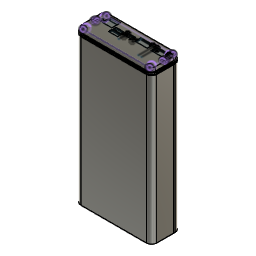
PowerBank65W v5 (Autodesk Fusion 360 design; units mm, degrees)
Autodesk Fusion 360 part; units mm, degrees
sketch "Sketch1" plane through (0, 0, 0) normal (0, 0, 1) x (1, 0, 0) in component "PWRBankModule"
  line L0 (3, 0) -> (78, 0)
  line L1 (81, 3) -> (81, 24)
  line L2 (78, 27) -> (3, 27)
  line L3 (0, 24) -> (0, 3)
  line L4 (2, 0) -> (2, 14.5)
  line L5 (2, 14.5) -> (0, 14.5)
  line L6 (0, 16.5) -> (2, 16.5)
  line L7 (2, 16.5) -> (2, 27)
  line L8 (79, 0) -> (79, 14.5)
  line L9 (79, 14.5) -> (81, 14.5)
  line L10 (81, 16.5) -> (79, 16.5)
  line L11 (79, 16.5) -> (79, 27)
  arc A0 (3, 27) -> (0, 24) centre (3, 24) ccw
  arc A1 (0, 3) -> (3, 0) centre (3, 3) ccw
  arc A2 (78, 0) -> (81, 3) centre (78, 3) ccw
  arc A3 (81, 24) -> (78, 27) centre (78, 24) ccw
  line L12 (82.5, 3) -> (82.5, 24)
  arc A4 (82.5, 24) -> (78, 28.5) centre (78, 24) ccw
  line L13 (78, 28.5) -> (3, 28.5)
  arc A5 (3, 28.5) -> (-1.5, 24) centre (3, 24) ccw
  line L14 (-1.5, 24) -> (-1.5, 3)
  arc A6 (-1.5, 3) -> (3, -1.5) centre (3, 3) ccw
  line L15 (3, -1.5) -> (78, -1.5)
  arc A7 (78, -1.5) -> (82.5, 3) centre (78, 3) ccw
  point P0 (81, 0)
  point P1 (0, 27)
  dimension "d1" = 81
  dimension "d2" = 1.5
  dimension "d3" = 77
  dimension "d4" = 2
  dimension "d5" = 2
  dimension "d6" = 2
  dimension "d7" = 2
  dimension "d8" = 2
  dimension "d9" = 14.5
  dimension "d10" = 14.5
  dimension "d11" = 27
  dimension "d50" = 3
  dimension "d51" = 3
  dimension "d52" = 3
  dimension "d53" = 3
  dimension "d54" = 12.5
  constraint horizontal L0
  constraint vertical L1
  constraint horizontal L2
  constraint vertical L3
  constraint coincident L0 L4.start
  constraint perpendicular L0 L4
  constraint coincident L3 L5.end
  constraint perpendicular L3 L5
  constraint coincident L3 L6.start
  constraint perpendicular L3 L6
  constraint coincident L2 L7.end
  constraint perpendicular L2 L7
  constraint coincident L0 L8.start
  constraint perpendicular L0 L8
  constraint coincident L1 L9.end
  constraint perpendicular L1 L9
  constraint coincident L1 L10.start
  constraint perpendicular L1 L10
  constraint coincident L2 L11.end
  constraint perpendicular L2 L11
  constraint coincident P1 L2
  constraint coincident P1 L3
  constraint tangent L2 A0
  constraint tangent L3 A0
  constraint coincident origin L0
  constraint coincident origin L3
  constraint tangent L0 A1
  constraint tangent L3 A1
  constraint coincident P0 L0
  constraint coincident P0 L1
  constraint tangent L0 A2
  constraint tangent L1 A2
  constraint tangent L1 A3
  constraint tangent L2 A3
  measures "d1" distance of origin P0
  measures "d3" distance of L4 L8
  measures "d4" distance of L4.end L5.end
  measures "d5" distance of L6.start L6.end
  measures "d6" distance of L10.start L10.end
  measures "d7" distance of L5 L6
  measures "d8" distance of L9 L10
  measures "d9" distance of L8.start L8.end
  measures "d10" distance of L4.start L4.end
  measures "d11" distance of origin P1
  measures "d50" radius of A0
  measures "d51" radius of A1
  measures "d52" radius of A2
  measures "d53" radius of A3
  measures "d54" distance of L2 L5
extrude "Extrude1" add sketch "Sketch1" along normal blind 3 contours L3 L4 L5 A1 | L1 L8 L9 A2 | L3 L6 L7 A0 | L1 L10 L11 A3 | L12 A4 L13 A5 L14 A6 L15 A7 makes body 1 in component "PWRBankModule"
sketch "Sketch2" plane through (0, 0, 3) normal (0, 0, 1) x (-1, 0, 0) in component "PWRBankModule"
  line L0 (-78, 0) -> (-3, 0)
  line L1 (0, -14.5) -> (0, -16.5)
  line L2 (-3, -27) -> (-78, -27)
  line L3 (-81, -16.5) -> (-81, -14.5)
  line L4 (-3, 1.5) -> (-78, 1.5)
  line L5 (-82.5, -3) -> (-82.5, -24)
  line L6 (-78, -28.5) -> (-3, -28.5)
  line L7 (1.5, -24) -> (1.5, -3)
  line L8 (-78, 0) -> (-3, 0) construction
  line L9 (-2, -0.1716) -> (-2, -14.5) construction
  line L10 (-2, -14.5) -> (0, -14.5) construction
  line L11 (0, -14.5) -> (0, -16.5) construction
  line L12 (0, -16.5) -> (-2, -16.5) construction
  line L13 (-2, -16.5) -> (-2, -26.8284) construction
  line L14 (-3, -27) -> (-78, -27) construction
  line L15 (-81, -16.5) -> (-81, -14.5) construction
  line L16 (-81, -14.5) -> (-79, -14.5) construction
  line L17 (-79, -14.5) -> (-79, -0.1716) construction
  line L18 (-79, -26.8284) -> (-79, -16.5) construction
  line L19 (-79, -16.5) -> (-81, -16.5) construction
  line L20 (-64, -23.1) -> (-78, -23.1)
  line L21 (-78, -23.1) -> (-78, -16.5)
  line L22 (-78, -16.5) -> (-64, -16.5)
  line L23 (-64, -16.5) -> (-64, -23.1)
  line L24 (-45.5, -23.1) -> (-59.5, -23.1)
  line L25 (-59.5, -23.1) -> (-59.5, -16.5)
  line L26 (-59.5, -16.5) -> (-45.5, -16.5)
  line L27 (-45.5, -16.5) -> (-45.5, -23.1)
  line L28 (-33, -20.5) -> (-42.5, -20.5)
  line L29 (-42.5, -20.5) -> (-42.5, -16.5)
  line L30 (-42.5, -16.5) -> (-33, -16.5)
  line L31 (-33, -16.5) -> (-33, -20.5)
  line L32 (-21, -19.3) -> (-30, -19.3)
  line L33 (-30, -19.3) -> (-30, -16)
  line L34 (-30, -16) -> (-21, -16)
  line L35 (-21, -16) -> (-21, -19.3)
  line L36 (-20.5, -15) -> (-31, -15)
  line L37 (-31, -15) -> (-31, -11)
  line L38 (-31, -11) -> (-20.5, -11)
  line L39 (-20.5, -11) -> (-20.5, -15)
  line L40 (-8, -26.5) -> (-19, -26.5)
  line L41 (-19, -26.5) -> (-19, -16.5)
  line L42 (-19, -16.5) -> (-8, -16.5)
  line L43 (-8, -16.5) -> (-8, -26.5)
  circle A0 centre (-5.5, -18.5) radius 1.75
  arc A1 (-3, -27) -> (-2, -26.8284) centre (-3, -24) ccw
  arc A2 (-79, -26.8284) -> (-78, -27) centre (-78, -24) ccw
  arc A3 (-78, 0) -> (-79, -0.1716) centre (-78, -3) ccw
  arc A4 (-2, -0.1716) -> (-3, 0) centre (-3, -3) ccw
  arc A5 (-78, 1.5) -> (-82.5, -3) centre (-78, -3) ccw
  arc A6 (-82.5, -24) -> (-78, -28.5) centre (-78, -24) ccw
  arc A7 (-3, -28.5) -> (1.5, -24) centre (-3, -24) ccw
  arc A8 (1.5, -3) -> (-3, 1.5) centre (-3, -3) ccw
  line L44 (-2, -0.1716) -> (-2, -14.5)
  line L45 (-2, -14.5) -> (0, -14.5)
  line L46 (0, -16.5) -> (-2, -16.5)
  line L47 (-2, -16.5) -> (-2, -26.8284)
  line L48 (-79, -26.8284) -> (-79, -16.5)
  line L49 (-79, -16.5) -> (-81, -16.5)
  line L50 (-81, -14.5) -> (-79, -14.5)
  line L51 (-79, -14.5) -> (-79, -0.1716)
  dimension "d14" = 81
  dimension "d15" = 14
  dimension "d16" = 14
  dimension "d17" = 4.5
  dimension "d18" = 6.6
  dimension "d20" = 3
  dimension "d21" = 48
  dimension "d22" = 9.5
  dimension "d23" = 60
  dimension "d24" = 9
  dimension "d25" = 3.3
  dimension "d26" = 4
  dimension "d27" = 60.5
  dimension "d28" = 10.5
  dimension "d29" = 4
  dimension "d30" = 73
  dimension "d31" = 11
  dimension "d32" = 10
  dimension "d33" = 75.5
  dimension "d34" = 3.5
  dimension "d35" = 8.6
  dimension "d38" = 1.5
  dimension "d39" = 0.5
  dimension "d40" = 2
  dimension "d55" = 6.6
  dimension "d56" = 4
  dimension "d57" = 6.6
  dimension "d58" = 2
  constraint horizontal L20
  constraint vertical L21
  constraint horizontal L22
  constraint vertical L23
  constraint horizontal L24
  constraint vertical L25
  constraint horizontal L26
  constraint vertical L27
  constraint horizontal L28
  constraint vertical L29
  constraint horizontal L30
  constraint vertical L31
  constraint horizontal L32
  constraint vertical L33
  constraint horizontal L34
  constraint vertical L35
  constraint horizontal L36
  constraint vertical L37
  constraint horizontal L38
  constraint vertical L39
  constraint horizontal L40
  constraint vertical L41
  constraint horizontal L42
  constraint vertical L43
  measures "d14" distance of L11 L15
  measures "d15" distance of L20.start L20.end
  measures "d16" distance of L24.start L24.end
  measures "d17" distance of L23 L25
  measures "d18" distance of L20.end L21.end
  measures "d20" distance of L15 L21
  measures "d21" distance of L15 L31
  measures "d22" distance of L28.start L28.end
  measures "d23" distance of L3 L35
  measures "d24" distance of L32.start L32.end
  measures "d25" distance of L32.end L33.end
  measures "d26" distance of L28.start L30.end
  measures "d27" distance of L15 L39
  measures "d28" distance of L36.start L36.end
  measures "d29" distance of L36.end L37.end
  measures "d30" distance of L15 L43
  measures "d31" distance of L40.start L40.end
  measures "d32" distance of L40.start L42.end
  measures "d33" distance of L15 A0.centre
  measures "d34" diameter of A0
  measures "d35" distance of L16 L20
  measures "d38" distance of L16 L34
  measures "d39" distance of L16 L36
  measures "d40" distance of L16 L42
  measures "d55" distance of L19 L24
  measures "d56" distance of L28 L49
  measures "d57" distance of L24.end L25.end
  measures "d58" distance of A0.centre L49
extrude "Extrude2" add sketch "Sketch2" along normal blind 1.5 contours L0 L1 L2 L3 A1 A2 A3 A4 L44 L45 L46 L47 L48 L49 L50 L51 | L4 L5 L6 L7 A5 A6 A7 A8 bodies 1 in component "PWRBankModule"
sketch "Sketch3" plane through (0, 0, 3) normal (0, 0, -1) x (1, 0, 0) in component "PWRBankModule"
  line L0 (45.5, -16.5) -> (59.5, -16.5)
  line L1 (59.5, -16.5) -> (59.5, -23.1)
  line L2 (59.5, -23.1) -> (45.5, -23.1)
  line L3 (45.5, -23.1) -> (45.5, -16.5)
  line L4 (33, -16.5) -> (42.5, -16.5)
  line L5 (42.5, -16.5) -> (42.5, -20.5)
  line L6 (42.5, -20.5) -> (33, -20.5)
  line L7 (33, -20.5) -> (33, -16.5)
  line L8 (64, -16.5) -> (78, -16.5)
  line L9 (78, -16.5) -> (78, -23.1)
  line L10 (78, -23.1) -> (64, -23.1)
  line L11 (64, -23.1) -> (64, -16.5)
  line L12 (21, -16) -> (30, -16)
  line L13 (30, -16) -> (30, -19.3)
  line L14 (30, -19.3) -> (21, -19.3)
  line L15 (21, -19.3) -> (21, -16)
  line L16 (20.5, -11) -> (31, -11)
  line L17 (31, -11) -> (31, -15)
  line L18 (31, -15) -> (20.5, -15)
  line L19 (20.5, -15) -> (20.5, -11)
  circle A0 centre (5.5, -18.5) radius 1.75
  line L20 (8, -16.5) -> (19, -16.5)
  line L21 (19, -16.5) -> (19, -26.5)
  line L22 (19, -26.5) -> (8, -26.5)
  line L23 (8, -26.5) -> (8, -16.5)
  line L24 (78, -23.1) -> (45.4821, -23.1)
  line L25 (45.4821, -23.1) -> (45.4821, -24.1)
  line L26 (45.4821, -24.1) -> (78, -24.1)
  line L27 (78, -24.1) -> (78, -23.1)
  line L28 (64, -23.1) -> (63, -23.1)
  line L29 (63, -23.1) -> (63, -6)
  line L30 (63, -6) -> (64, -6)
  line L31 (64, -6) -> (64, -23.1)
  line L32 (59.5, -23.1) -> (60.5, -23.1)
  line L33 (60.5, -23.1) -> (60.5, -6)
  line L34 (60.5, -6) -> (59.5, -6)
  line L35 (59.5, -6) -> (59.5, -23.1)
  line L36 (33, -20.5) -> (43.5, -20.5)
  line L37 (43.5, -20.5) -> (43.5, -21.5)
  line L38 (43.5, -21.5) -> (33, -21.5)
  line L39 (33, -21.5) -> (33, -20.5)
  line L40 (43.5, -20.5) -> (42.5, -20.5)
  line L41 (42.5, -20.5) -> (42.5, -16.5)
  line L42 (42.5, -16.5) -> (43.5, -16.5)
  line L43 (43.5, -16.5) -> (43.5, -20.5)
  line L44 (33, -16.5) -> (32, -16.5)
  line L45 (32, -16.5) -> (32, -10.9)
  line L46 (32, -10.9) -> (33, -10.9)
  line L47 (33, -10.9) -> (33, -16.5)
  line L48 (78, 0) -> (3, 0)
  arc A1 (3, 0) -> (2, -0.1716) centre (3, -3) ccw
  line L49 (2, -0.1716) -> (2, -14.5)
  line L50 (2, -14.5) -> (0, -14.5)
  line L51 (0, -14.5) -> (0, -16.5)
  line L52 (0, -16.5) -> (2, -16.5)
  line L53 (2, -16.5) -> (2, -26.8284)
  arc A2 (2, -26.8284) -> (3, -27) centre (3, -24) ccw
  line L54 (3, -27) -> (78, -27)
  arc A3 (78, -27) -> (79, -26.8284) centre (78, -24) ccw
  line L55 (79, -26.8284) -> (79, -16.5)
  line L56 (79, -16.5) -> (81, -16.5)
  line L57 (81, -16.5) -> (81, -14.5)
  line L58 (81, -14.5) -> (79, -14.5)
  line L59 (79, -14.5) -> (79, -0.1716)
  arc A4 (79, -0.1716) -> (78, 0) centre (78, -3) ccw
  dimension "d44" = 1
  dimension "d45" = 1
  dimension "d46" = 1
  dimension "d47" = 1
  dimension "d48" = 1
  dimension "d49" = 1
  constraint horizontal L24
  constraint vertical L25
  constraint horizontal L26
  constraint vertical L27
  constraint coincident L9.end L10.start
  constraint horizontal L28
  constraint vertical L29
  constraint horizontal L30
  constraint vertical L31
  constraint coincident L10.end L11.start
  constraint horizontal L32
  constraint vertical L33
  constraint horizontal L34
  constraint vertical L35
  constraint coincident L1.end L2.start
  constraint horizontal L36
  constraint vertical L37
  constraint horizontal L38
  constraint vertical L39
  constraint coincident L6.end L7.start
  constraint horizontal L40
  constraint vertical L41
  constraint horizontal L42
  constraint vertical L43
  constraint coincident L4.end L5.start
  constraint horizontal L44
  constraint vertical L45
  constraint horizontal L46
  constraint vertical L47
  constraint coincident L4.start L7.end
  measures "d44" distance of L9.end L26.end
  measures "d45" distance of L29.end L30.end
  measures "d46" distance of L33.end L34.end
  measures "d47" distance of L36.end L37.end
  measures "d48" distance of L4.end L42.end
  measures "d49" distance of L4.start L44.end
sketch "Sketch1 (2)" plane through (0, 0, 0) normal (0, 0, 1) x (1, 0, 0) in component "ButtLid"
  line L0 (3, -1.5) -> (78, -1.5) construction
  arc A0 (78, -1.5) -> (82.5, 3) centre (78, 3) ccw construction
  line L1 (82.5, 3) -> (82.5, 24) construction
  arc A1 (82.5, 24) -> (78, 28.5) centre (78, 24) ccw construction
  line L2 (78, 28.5) -> (3, 28.5) construction
  arc A2 (3, 28.5) -> (-1.5, 24) centre (3, 24) ccw construction
  line L3 (-1.5, 24) -> (-1.5, 3) construction
  arc A3 (-1.5, 3) -> (3, -1.5) centre (3, 3) ccw construction
  arc A4 (3, 28.6) -> (-1.6, 24) centre (3, 24) ccw
  line L4 (-1.6, 24) -> (-1.6, 3)
  arc A5 (-1.6, 3) -> (3, -1.6) centre (3, 3) ccw
  line L5 (3, -1.6) -> (78, -1.6)
  arc A6 (78, -1.6) -> (82.6, 3) centre (78, 3) ccw
  line L6 (82.6, 3) -> (82.6, 24)
  arc A7 (82.6, 24) -> (78, 28.6) centre (78, 24) ccw
  line L7 (78, 28.6) -> (3, 28.6)
  arc A8 (3, 30) -> (-3, 24) centre (3, 24) ccw
  line L8 (-3, 24) -> (-3, 3)
  arc A9 (-3, 3) -> (3, -3) centre (3, 3) ccw
  line L9 (3, -3) -> (78, -3)
  arc A10 (78, -3) -> (84, 3) centre (78, 3) ccw
  line L10 (84, 3) -> (84, 24)
  arc A11 (84, 24) -> (78, 30) centre (78, 24) ccw
  line L11 (78, 30) -> (3, 30)
  line L12 (84, 22) -> (82.6, 22)
  line L13 (82.6, 21) -> (81.1, 21)
  line L14 (81.1, 21) -> (81.1, 23)
  line L15 (81.1, 23) -> (82.5, 23)
  line L16 (82.5, 23) -> (82.5, 22)
  line L17 (82.5, 22) -> (82.6, 22)
  line L18 (-1.6, 22) -> (-3, 22)
  line L19 (-1.6, 22) -> (-1.5, 22)
  line L20 (-1.5, 22) -> (-1.5, 23)
  line L21 (-1.5, 23) -> (-0.1, 23)
  line L22 (-0.1, 23) -> (-0.1, 21)
  line L23 (-0.1, 21) -> (-1.6, 21)
  dimension "d59" = 0.1
  dimension "d60" = 1.5
  dimension "d61" = 1
  dimension "d62" = 2
  dimension "d63" = 1.5
  dimension "d64" = 0.1
  dimension "d65" = 25
  dimension "d70" = 1.5
  dimension "d71" = 2
  dimension "d72" = 1
  dimension "d73" = 0.1
  dimension "d74" = 25
  constraint coincident L6 L12.end
  constraint perpendicular L6 L12
  constraint coincident L6 L13.start
  constraint perpendicular L1 L13
  constraint perpendicular L13 L14
  constraint perpendicular L14 L15
  constraint perpendicular L15 L16
  constraint perpendicular L6 L17
  constraint coincident L4 L18.start
  constraint coincident L8 L18.end
  constraint perpendicular L8 L18
  constraint perpendicular L3 L19
  constraint perpendicular L18 L20
  constraint perpendicular L3 L21
  constraint perpendicular L21 L22
  constraint coincident L4 L23.end
  constraint perpendicular L4 L23
  measures "d61" distance of L15.end L16.end
  measures "d62" distance of L13.end L14.end
  measures "d63" distance of L13.start L13.end
  measures "d64" distance of L6 L16
  measures "d65" distance of L9 L12
  measures "d70" distance of L22.end L23.end
  measures "d71" distance of L21.end L22.end
  measures "d72" distance of L19.end L20.end
  measures "d73" distance of L18.start L19.end
  measures "d74" distance of L9 L18
extrude "Extrude1'" add sketch "Sketch1 (2)" against normal blind 170 separate body contours L4 L19 L20 L21 L22 L23 | L4 A5 L5 A6 L6 L8 A9 L9 A10 L10 L12 L18 | L6 L13 L14 L15 L16 L17 makes body 2 in component "ButtLid"
sketch "Sketch2 (2)" plane through (0, 0, 0) normal (0, 0, 1) x (-1, 0, 0) in component "ButtLid"
  line L0 (1.5, -22) -> (3, -22)
  line L1 (3, -22) -> (3, -3)
  arc A0 (3, -3) -> (-3, 3) centre (-3, -3) ccw
  line L2 (-3, 3) -> (-78, 3)
  arc A1 (-78, 3) -> (-84, -3) centre (-78, -3) ccw
  line L3 (-84, -3) -> (-84, -22)
  line L4 (-84, -22) -> (-82.5, -22)
  line L5 (-82.5, -22) -> (-82.5, -23)
  line L6 (-82.5, -23) -> (-81.1, -23)
  line L7 (-81.1, -23) -> (-81.1, -21)
  line L8 (-81.1, -21) -> (-82.6, -21)
  line L9 (-82.6, -21) -> (-82.6, -3)
  arc A2 (-78, 1.6) -> (-82.6, -3) centre (-78, -3) ccw
  line L10 (-78, 1.6) -> (-3, 1.6)
  arc A3 (1.6, -3) -> (-3, 1.6) centre (-3, -3) ccw
  line L11 (1.6, -3) -> (1.6, -21)
  line L12 (1.6, -21) -> (0.1, -21)
  line L13 (0.1, -21) -> (0.1, -23)
  line L14 (0.1, -23) -> (1.5, -23)
  line L15 (1.5, -23) -> (1.5, -22)
  line L16 (-82.6, -17.5) -> (-79, -17.5)
  line L17 (-79, -17.5) -> (-79, -16.5)
  line L18 (-79, -16.5) -> (-81, -16.5)
  line L19 (-81, -16.5) -> (-81, -14.5)
  line L20 (-81, -14.5) -> (-79, -14.5)
  line L21 (-79, -14.5) -> (-79, -13.5)
  line L22 (-79, -13.5) -> (-82.6, -13.5)
  line L23 (1.6, -17.5) -> (-2, -17.5)
  line L24 (-2, -17.5) -> (-2, -16.5)
  line L25 (-2, -16.5) -> (0, -16.5)
  line L26 (0, -16.5) -> (0, -14.5)
  line L27 (0, -14.5) -> (-2, -14.5)
  line L28 (-2, -14.5) -> (-2, -13.5)
  line L29 (-2, -13.5) -> (1.6, -13.5)
  point P0 (-79, -16.5)
  point P1 (-81, -16.5)
  point P2 (-81, -14.5)
  point P3 (-79, -14.5)
  point P4 (0, -14.5)
  point P5 (-2, -14.5)
  point P6 (-2, -16.5)
  point P7 (0, -16.5)
  dimension "d77" = 1
  dimension "d78" = 1
  dimension "d79" = 1
  dimension "d80" = 1
  constraint coincident L9 L16.start
  constraint perpendicular L9 L16
  constraint coincident P0 L17.end
  constraint coincident P1 L18.end
  constraint coincident P2 L19.end
  constraint coincident P3 L20.end
  constraint perpendicular L20 L21
  constraint coincident L9 L22.end
  constraint perpendicular L9 L22
  constraint coincident L11 L23.start
  constraint perpendicular L11 L23
  constraint coincident P6 L24.end
  constraint coincident P7 L25.end
  constraint coincident P4 L26.end
  constraint coincident P5 L27.end
  constraint perpendicular L27 L28
  constraint coincident L11 L29.end
  constraint perpendicular L11 L29
  measures "d77" distance of L16.end P0
  measures "d78" distance of P3 L21.end
  measures "d79" distance of P5 L28.end
  measures "d80" distance of L23.end P6
extrude "Extrude2'" add sketch "Sketch2 (2)" against normal blind 28 contours L11 L23 L24 L25 L26 L27 L28 L29 | L9 L16 L17 L18 L19 L20 L21 L22 bodies 2 in component "ButtLid"
sketch "Sketch3 (2)" plane through (0, 0, 0) normal (0, 0, 1) x (-1, 0, 0) in component "ButtLid"
  line L0 (1.5, -22) -> (3, -22)
  line L1 (3, -22) -> (3, -3)
  arc A0 (3, -3) -> (-3, 3) centre (-3, -3) ccw
  line L2 (-3, 3) -> (-78, 3)
  arc A1 (-78, 3) -> (-84, -3) centre (-78, -3) ccw
  line L3 (-84, -3) -> (-84, -22)
  line L4 (-84, -22) -> (-82.5, -22)
  line L5 (-82.5, -22) -> (-82.5, -23)
  line L6 (-82.5, -23) -> (-81.1, -23)
  line L7 (-81.1, -23) -> (-81.1, -21)
  line L8 (-81.1, -21) -> (-82.6, -21)
  line L9 (-82.6, -21) -> (-82.6, -17.5)
  line L10 (-82.6, -17.5) -> (-79, -17.5)
  line L11 (-79, -17.5) -> (-79, -16.5)
  line L12 (-79, -16.5) -> (-81, -16.5)
  line L13 (-81, -16.5) -> (-81, -14.5)
  line L14 (-81, -14.5) -> (-79, -14.5)
  line L15 (-79, -14.5) -> (-79, -13.5)
  line L16 (-79, -13.5) -> (-82.6, -13.5)
  line L17 (-82.6, -13.5) -> (-82.6, -3)
  arc A2 (-78, 1.6) -> (-82.6, -3) centre (-78, -3) ccw
  line L18 (-78, 1.6) -> (-3, 1.6)
  arc A3 (1.6, -3) -> (-3, 1.6) centre (-3, -3) ccw
  line L19 (1.6, -3) -> (1.6, -13.5)
  line L20 (1.6, -13.5) -> (-2, -13.5)
  line L21 (-2, -13.5) -> (-2, -14.5)
  line L22 (-2, -14.5) -> (0, -14.5)
  line L23 (0, -14.5) -> (0, -16.5)
  line L24 (0, -16.5) -> (-2, -16.5)
  line L25 (-2, -16.5) -> (-2, -17.5)
  line L26 (-2, -17.5) -> (1.6, -17.5)
  line L27 (1.6, -17.5) -> (1.6, -21)
  line L28 (1.6, -21) -> (0.1, -21)
  line L29 (0.1, -21) -> (0.1, -23)
  line L30 (0.1, -23) -> (1.5, -23)
  line L31 (1.5, -23) -> (1.5, -22)
  line L32 (-82.6, -13.5) -> (-79, -13.5)
  line L33 (-79, -13.5) -> (-79, -23)
  line L34 (-79, -23) -> (-82.6, -23)
  line L35 (-82.6, -23) -> (-82.6, -13.5)
  line L36 (1.6, -13.5) -> (-2, -13.5)
  line L37 (-2, -13.5) -> (-2, -23)
  line L38 (-2, -23) -> (1.6, -23)
  line L39 (1.6, -23) -> (1.6, -13.5)
  dimension "d83" = 3.6
  dimension "d84" = 3.6
  constraint horizontal L32
  constraint vertical L33
  constraint horizontal L34
  constraint vertical L35
  constraint coincident L16.end L17.start
  constraint horizontal L36
  constraint vertical L37
  constraint horizontal L38
  constraint vertical L39
  constraint coincident L19.end L20.start
  constraint coincident L6.end L34
  constraint coincident L29.end L38
  measures "d83" distance of L33.end L34.end
  measures "d84" distance of L37.end L38.end
extrude "Extrude3" cut sketch "Sketch3 (2)" against normal blind 4.6 contours L0 L28 L29 L30 L31 L38 L39 | L20 L21 L22 L23 L24 L25 L26 L36 L37 L39 | L4 L5 L6 L7 L8 L34 L35 | L10 L11 L12 L13 L14 L15 L16 L32 L33 L35 bodies 2 in component "ButtLid"
sketch "Sketch4" plane through (0, 0, -170) normal (0, 0, -1) x (1, 0, 0) in component "ButtLid"
  line L0 (-3, -22) -> (-1.5, -22)
  line L1 (-1.5, -22) -> (-1.5, -23)
  line L2 (-1.5, -23) -> (-0.1, -23)
  line L3 (-0.1, -23) -> (-0.1, -21)
  line L4 (-0.1, -21) -> (-1.6, -21)
  line L5 (-1.6, -21) -> (-1.6, -3)
  arc A0 (3, 1.6) -> (-1.6, -3) centre (3, -3) ccw
  line L6 (3, 1.6) -> (78, 1.6)
  arc A1 (82.6, -3) -> (78, 1.6) centre (78, -3) ccw
  line L7 (82.6, -3) -> (82.6, -21)
  line L8 (82.6, -21) -> (81.1, -21)
  line L9 (81.1, -21) -> (81.1, -23)
  line L10 (81.1, -23) -> (82.5, -23)
  line L11 (82.5, -23) -> (82.5, -22)
  line L12 (82.5, -22) -> (84, -22)
  line L13 (84, -22) -> (84, -3)
  arc A2 (84, -3) -> (78, 3) centre (78, -3) ccw
  line L14 (78, 3) -> (3, 3)
  arc A3 (3, 3) -> (-3, -3) centre (3, -3) ccw
  line L15 (-3, -3) -> (-3, -22)
  line L16 (-1.6, -21) -> (-0.1, -21)
  line L17 (-0.1, -21) -> (-0.1, -23)
  line L18 (-0.1, -23) -> (-1.6, -23)
  line L19 (-1.6, -23) -> (-1.6, -21)
  line L20 (82.6, -21) -> (81.1, -21)
  line L21 (81.1, -21) -> (81.1, -23)
  line L22 (81.1, -23) -> (82.6, -23)
  line L23 (82.6, -23) -> (82.6, -21)
  constraint horizontal L16
  constraint vertical L17
  constraint horizontal L18
  constraint vertical L19
  constraint coincident L2.end L3.start
  constraint coincident L4.end L5.start
  constraint horizontal L20
  constraint vertical L21
  constraint horizontal L22
  constraint vertical L23
  constraint coincident L9.end L10.start
  constraint coincident L7.end L8.start
extrude "Extrude4" cut sketch "Sketch4" against normal blind 1.6 contours L0 L1 L2 L3 L4 L16 L17 L18 L19 | L8 L9 L10 L11 L12 L20 L21 L22 L23 bodies 2 in component "ButtLid"
sketch "Sketch1 (3)" plane through (0, 0, 0) normal (0, 0, -1) x (1, 0, 0) in component "TopLid"
  arc A0 (3, 0) -> (2, -0.1716) centre (3, -3) ccw
  line L0 (3, 0) -> (78, 0)
  arc A1 (79, -0.1716) -> (78, 0) centre (78, -3) ccw
  line L1 (79, -0.1716) -> (79, -14.5)
  line L2 (79, -14.5) -> (81, -14.5)
  line L3 (81, -14.5) -> (81, -16.5)
  line L4 (81, -16.5) -> (79, -16.5)
  line L5 (79, -16.5) -> (79, -26.8284)
  arc A2 (78, -27) -> (79, -26.8284) centre (78, -24) ccw
  line L6 (78, -27) -> (3, -27)
  arc A3 (2, -26.8284) -> (3, -27) centre (3, -24) ccw
  line L7 (2, -26.8284) -> (2, -16.5)
  line L8 (2, -16.5) -> (0, -16.5)
  line L9 (0, -16.5) -> (0, -14.5)
  line L10 (0, -14.5) -> (2, -14.5)
  line L11 (2, -14.5) -> (2, -0.1716)
  arc A4 (82.5, -3) -> (78, 1.5) centre (78, -3) ccw
  line L12 (78, 1.5) -> (3, 1.5)
  arc A5 (3, 1.5) -> (-1.5, -3) centre (3, -3) ccw
  line L13 (-1.5, -3) -> (-1.5, -24)
  arc A6 (-1.5, -24) -> (3, -28.5) centre (3, -24) ccw
  line L14 (3, -28.5) -> (78, -28.5)
  arc A7 (78, -28.5) -> (82.5, -24) centre (78, -24) ccw
  line L15 (82.5, -24) -> (82.5, -3)
  line L16 (78, -28.5) -> (3, -28.5) construction
  arc A8 (-1.5, -24) -> (3, -28.5) centre (3, -24) ccw construction
  line L17 (-1.5, -24) -> (-1.5, -3) construction
  line L18 (-3, -22) -> (-1.6, -22) construction
  arc A9 (78, -28.5) -> (82.5, -24) centre (78, -24) ccw construction
  line L19 (82.5, -3) -> (82.5, -24) construction
  line L20 (82.6, -22) -> (84, -22) construction
  arc A10 (82.6, -3) -> (78, 1.6) centre (78, -3) ccw
  line L21 (78, 1.6) -> (3, 1.6)
  arc A11 (3, 1.6) -> (-1.6, -3) centre (3, -3) ccw
  line L22 (-1.6, -3) -> (-1.6, -24)
  arc A12 (-1.6, -24) -> (3, -28.6) centre (3, -24) ccw
  line L23 (3, -28.6) -> (78, -28.6)
  arc A13 (78, -28.6) -> (82.6, -24) centre (78, -24) ccw
  line L24 (82.6, -24) -> (82.6, -3)
  arc A14 (84, -3) -> (78, 3) centre (78, -3) ccw
  line L25 (78, 3) -> (3, 3)
  arc A15 (3, 3) -> (-3, -3) centre (3, -3) ccw
  line L26 (-3, -3) -> (-3, -24)
  arc A16 (-3, -24) -> (3, -30) centre (3, -24) ccw
  line L27 (3, -30) -> (78, -30)
  arc A17 (78, -30) -> (84, -24) centre (78, -24) ccw
  line L28 (84, -24) -> (84, -3)
  line L29 (84, -21.9) -> (82.6, -21.9)
  line L30 (-1.6, -21.9) -> (-3, -21.9)
  dimension "d89" = 0.1
  dimension "d90" = 1.5
  dimension "d101" = 0.1
  dimension "d102" = 0.1
  constraint coincident L28 L29.start
  constraint coincident L24 L29.end
  constraint perpendicular L24 L29
  constraint coincident L22 L30.start
  constraint coincident L26 L30.end
  constraint perpendicular L26 L30
  measures "d101" distance of L18 L30
  measures "d102" distance of L20 L29
extrude "Extrude1''" add sketch "Sketch1 (3)" along normal blind 170 separate body contours L22 A12 L23 A13 L24 L26 A16 L27 A17 L28 L29 L30 makes body 3 in component "TopLid"
sketch "Sketch2 (3)" plane through (0, 30, 0) normal (0, 1, 0) x (-1, 0, 0) in component "TopLid"
  line L0 (-3, 0) -> (-78, 0)
  line L1 (-78, 0) -> (-78, -170)
  line L2 (-78, -170) -> (-3, -170)
  line L3 (-3, -170) -> (-3, 0)
  line L4 (-32, -5) -> (-19, -5)
  line L5 (-19, -5) -> (-19, -14)
  line L6 (-19, -14) -> (-32, -14)
  line L7 (-32, -14) -> (-32, -5)
  line L8 (3, 0) -> (3, -170)
  dimension "d95" = 5
  dimension "d96" = 13
  dimension "d97" = 22
  dimension "d98" = 9
  constraint horizontal L4
  constraint vertical L5
  constraint horizontal L6
  constraint vertical L7
  measures "d95" distance of L0 L4
  measures "d96" distance of L5.end L6.end
  measures "d97" distance of L5 L8
  measures "d98" distance of L4.start L6.end
extrude "Extrude2''" cut sketch "Sketch2 (3)" against normal blind 1.5 contours L4 L5 L6 L7 bodies 3 in component "TopLid"
sketch "Sketch1 (4)" plane through (0, 0, 0) normal (0, 0, 1) x (1, 0, 0) in component "BackLid"
  line L0 (82.5, 3) -> (82.5, 24)
  arc A0 (82.5, 24) -> (78, 28.5) centre (78, 24) ccw
  line L1 (78, 28.5) -> (3, 28.5)
  arc A1 (78, -1.5) -> (82.5, 3) centre (78, 3) ccw
  line L2 (3, -1.5) -> (78, -1.5)
  arc A2 (-1.5, 3) -> (3, -1.5) centre (3, 3) ccw
  line L3 (-1.5, 24) -> (-1.5, 3)
  arc A3 (3, 28.5) -> (-1.5, 24) centre (3, 24) ccw
extrude "Extrude1'''" add sketch "Sketch1 (4)" against normal blind 1.5 separate body makes body 4 in component "BackLid"
sketch "Sketch2 (4)" plane through (0, 0, -1.5) normal (0, 0, -1) x (1, 0, 0) in component "BackLid"
  arc A0 (-1.5, -24) -> (3, -28.5) centre (3, -24) ccw
  line L0 (3, -28.5) -> (78, -28.5)
  arc A1 (78, -28.5) -> (82.5, -24) centre (78, -24) ccw
  line L1 (82.5, -24) -> (82.5, -3)
  arc A2 (82.5, -3) -> (78, 1.5) centre (78, -3) ccw
  line L2 (78, 1.5) -> (3, 1.5)
  arc A3 (3, 1.5) -> (-1.5, -3) centre (3, -3) ccw
  line L3 (-1.5, -3) -> (-1.5, -24)
  arc A4 (3, 3) -> (-3, -3) centre (3, -3) ccw
  line L4 (-3, -3) -> (-3, -24)
  arc A5 (-3, -24) -> (3, -30) centre (3, -24) ccw
  line L5 (3, -30) -> (78, -30)
  arc A6 (78, -30) -> (84, -24) centre (78, -24) ccw
  line L6 (84, -24) -> (84, -3)
  arc A7 (84, -3) -> (78, 3) centre (78, -3) ccw
  line L7 (78, 3) -> (3, 3)
  dimension "d105" = 1.5
extrude "Extrude2'''" add sketch "Sketch2 (4)" along normal blind 1 contours A0 L0 A1 L1 A2 L2 A3 L3 | A4 L4 A5 L5 A6 L6 A7 L7 bodies 4 in component "BackLid"
component "PWRBankModule" placed x (1, 0, 0) y (0, 1, 0) z (0, 0, 1) at (0, 0, 0)
component "ButtLid" placed x (1, 0, 0) y (0, 1, 0) z (0, 0, 1) at (0, 0, 0)
component "TopLid" placed x (1, 0, 0) y (0, 1, 0) z (0, 0, 1) at (0, 0, 0)
component "BackLid" placed x (1, 0, 0) y (0, 1, 0) z (0, 0, 1) at (0, 0, 0)
